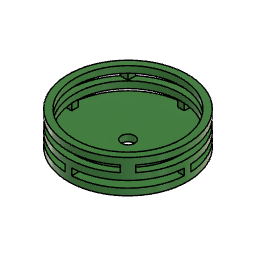
Spring_11 mm h_v5 v2 (Autodesk Fusion 360 design; units mm, degrees)
Autodesk Fusion 360 part; units mm, degrees
sketch "Sketch1" plane through (0, 0, 0) normal (0, 0, 1) x (1, 0, 0)
  circle A0 centre (0, 0) radius 9
  circle A1 centre (0, 0) radius 1
  dimension "d1" = 18
  dimension "d2" = 2
  constraint concentric A0 A1
  constraint coincident A0.centre A1.centre
  measures "d1" diameter of A0
  measures "d2" diameter of A1
extrude "Extrude1" add sketch "Sketch1" along normal blind 11
ref_plane "WorkPlane1" through (0, -18, 0) normal (0, 1, 0) x (0, 0, 1)
sketch "Holes1" plane through (0, -18, 0) normal (0, 1, 0) x (1, 0, 0)
  line L0 (-8, -10) -> (-0.5, -10)
  line L1 (-0.5, -10) -> (-0.5, -9)
  line L2 (-0.5, -9) -> (-8, -9)
  line L3 (-8, -9) -> (-8, -10)
  line L4 (0.5, -10) -> (8, -10)
  line L5 (8, -9) -> (0.5, -9)
  line L6 (8, -10) -> (8, -9)
  line L7 (0.5, -9) -> (0.5, -10)
  line L8 (-8, -6) -> (-0.5, -6)
  line L9 (-0.5, -5) -> (-8, -5)
  line L10 (-0.5, -6) -> (-0.5, -5)
  line L11 (-8, -5) -> (-8, -6)
  line L12 (0.5, -6) -> (8, -6)
  line L13 (8, -5) -> (0.5, -5)
  line L14 (8, -6) -> (8, -5)
  line L15 (0.5, -5) -> (0.5, -6)
  line L16 (-8, -2) -> (-0.5, -2)
  line L17 (-0.5, -1) -> (-8, -1)
  line L18 (-0.5, -2) -> (-0.5, -1)
  line L19 (-8, -1) -> (-8, -2)
  line L20 (0.5, -2) -> (8, -2)
  line L21 (8, -1) -> (0.5, -1)
  line L22 (8, -2) -> (8, -1)
  line L23 (0.5, -1) -> (0.5, -2)
  line L24 (14.5287, -11) -> (-18, -11) construction
  line L25 (-9, -21) -> (-9, 10) construction
  line L26 (-5.75, -8) -> (5.75, -8)
  line L27 (5.75, -8) -> (5.75, -7)
  line L28 (5.75, -7) -> (-5.75, -7)
  line L29 (-5.75, -7) -> (-5.75, -8)
  line L30 (-5.75, -4) -> (5.75, -4)
  line L31 (5.75, -3) -> (-5.75, -3)
  line L32 (5.75, -4) -> (5.75, -3)
  line L33 (-5.75, -3) -> (-5.75, -4)
  dimension "d8" = 7.5
  dimension "d9" = 1
  dimension "d12" = 8.5
  dimension "d13" = 8
  dimension "d14" = 11
  dimension "d15" = 1
  dimension "d31" = 9
  dimension "d32" = 1
  dimension "d33" = 1
  dimension "d34" = 3.25
  dimension "d35" = 3
  dimension "d36" = 11.5
  dimension "d39" = 0
  dimension "d40" = 4
  constraint horizontal L0
  constraint vertical L1
  constraint horizontal L2
  constraint vertical L3
  constraint horizontal L24
  constraint vertical L25
  constraint horizontal L26
  constraint vertical L27
  constraint horizontal L28
  constraint vertical L29
  measures "d8" distance of L0.start L0.end
  measures "d9" distance of L0.start L2.end
  measures "d14" distance of origin L24
  measures "d15" distance of L0 L24
  measures "d31" distance of origin L25
  measures "d32" distance of L3 L25
  measures "d33" distance of L26.start L28.end
  measures "d34" distance of L25 L29
  measures "d35" distance of L24 L26
  measures "d36" distance of L26.start L26.end
extrude "Extrude2" cut sketch "Holes1" along normal blind 36
ref_plane "WorkPlane2" through (20, 0, 0) normal (1, 0, 0) x (0, 1, 0)
sketch "Holes2" plane through (20, 0, 0) normal (1, 0, 0) x (0, 1, 0)
  line L0 (-8, 10) -> (-0.5, 10)
  line L1 (-0.5, 10) -> (-0.5, 9)
  line L2 (-0.5, 9) -> (-8, 9)
  line L3 (-8, 9) -> (-8, 10)
  line L4 (-18.3444, 11) -> (18, 11) construction
  line L5 (0.5, 10) -> (8, 10)
  line L6 (8, 9) -> (0.5, 9)
  line L7 (8, 10) -> (8, 9)
  line L8 (0.5, 9) -> (0.5, 10)
  line L9 (-8, 6) -> (-0.5, 6)
  line L10 (-0.5, 5) -> (-8, 5)
  line L11 (-0.5, 6) -> (-0.5, 5)
  line L12 (-8, 5) -> (-8, 6)
  line L13 (0.5, 6) -> (8, 6)
  line L14 (8, 5) -> (0.5, 5)
  line L15 (8, 6) -> (8, 5)
  line L16 (0.5, 5) -> (0.5, 6)
  line L17 (-8, 2) -> (-0.5, 2)
  line L18 (-0.5, 1) -> (-8, 1)
  line L19 (-0.5, 2) -> (-0.5, 1)
  line L20 (-8, 1) -> (-8, 2)
  line L21 (0.5, 2) -> (8, 2)
  line L22 (8, 1) -> (0.5, 1)
  line L23 (8, 2) -> (8, 1)
  line L24 (0.5, 1) -> (0.5, 2)
  line L25 (-9, 15.6386) -> (-9, -5) construction
  line L26 (-5.75, 8) -> (5.75, 8)
  line L27 (5.75, 8) -> (5.75, 7)
  line L28 (5.75, 7) -> (-5.75, 7)
  line L29 (-5.75, 7) -> (-5.75, 8)
  line L30 (-5.75, 4) -> (5.75, 4)
  line L31 (5.75, 3) -> (-5.75, 3)
  line L32 (5.75, 4) -> (5.75, 3)
  line L33 (-5.75, 3) -> (-5.75, 4)
  dimension "d19" = 7.5
  dimension "d20" = 1
  dimension "d21" = 11
  dimension "d22" = 1
  dimension "d25" = 8.5
  dimension "d26" = -8
  dimension "d27" = 9
  dimension "d28" = 1
  dimension "d41" = 1
  dimension "d42" = 3
  dimension "d43" = 11.5
  dimension "d46" = 0
  dimension "d47" = -4
  dimension "d48" = 3.25
  constraint horizontal L0
  constraint vertical L1
  constraint horizontal L2
  constraint vertical L3
  constraint horizontal L4
  constraint vertical L25
  constraint horizontal L26
  constraint vertical L27
  constraint horizontal L28
  constraint vertical L29
  measures "d19" distance of L0.start L0.end
  measures "d20" distance of L0.start L2.end
  measures "d21" distance of origin L4
  measures "d22" distance of L0 L4
  measures "d27" distance of origin L25
  measures "d28" distance of L3 L25
  measures "d41" distance of L26.start L28.end
  measures "d42" distance of L4 L26
  measures "d43" distance of L26.start L26.end
  measures "d48" distance of L25 L29
extrude "Extrude3" cut sketch "Holes2" against normal blind 40
sketch "Hollow inside" plane through (0, 0, 1) normal (0, 0, 1) x (-1, 0, 0)
  line L0 (-0.5, 8) -> (-0.5, 8.9861)
  arc A0 (-0.5, 8.9861) -> (-8.9861, 0.5) centre (0, 0) ccw
  line L1 (-8.9861, 0.5) -> (-8, 0.5)
  line L2 (-8, 0.5) -> (-8, -0.5)
  line L3 (-8, -0.5) -> (-8.9861, -0.5)
  arc A1 (-8.9861, -0.5) -> (-0.5, -8.9861) centre (0, 0) ccw
  line L4 (-0.5, -8.9861) -> (-0.5, -8)
  line L5 (-0.5, -8) -> (0.5, -8)
  line L6 (0.5, -8) -> (0.5, -8.9861)
  arc A2 (0.5, -8.9861) -> (8.9861, -0.5) centre (0, 0) ccw
  line L7 (8.9861, -0.5) -> (8, -0.5)
  line L8 (8, -0.5) -> (8, 0.5)
  line L9 (8, 0.5) -> (8.9861, 0.5)
  arc A3 (8.9861, 0.5) -> (0.5, 8.9861) centre (0, 0) ccw
  line L10 (0.5, 8.9861) -> (0.5, 8)
  line L11 (0.5, 8) -> (-0.5, 8)
  circle A4 centre (0, 0) radius 8
  circle A5 centre (0, 0) radius 1
  dimension "d49" = 16
  constraint concentric A0 A4
  measures "d49" diameter of A4
extrude "Extrude4" cut sketch "Hollow inside" along normal up to surface (9 mm away) contours A4 | A5
sketch "Cut in half" plane through (0, 0, 5) normal (0, 0, 1) x (-1, 0, 0)
  arc A0 (0, -8) -> (8, 0) centre (0, 0) ccw
  line L0 (0, -8) -> (0.5, -8)
  line L1 (0.5, -8) -> (0.5, -8.9861)
  arc A1 (0.5, -8.9861) -> (8.9861, -0.5) centre (0, 0) ccw
  line L2 (8.9861, -0.5) -> (8, -0.5)
  line L3 (8, -0.5) -> (8, 0)
  circle A2 centre (0, 0) radius 9
  dimension "d52" = 18
  constraint coincident A0.centre A1.centre
  measures "d52" diameter of A2
extrude "Extrude5" cut sketch "Cut in half" along normal blind 11
